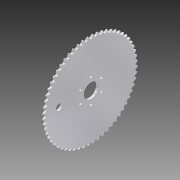
# Autodesk Inventor part: CatapultSprocket
Saved by Autodesk Inventor 2013 (Build 170138000, 138)
## iProperties
Category: iParts
Company: FirstCadLibrary
Shininess: 64.0
Length Units: 11272
Angle Units: 11279
Time Units: 11290
Mass Units: 11286
Length Display Precision: 3
Angle Display Precision: 2
Compacted: True
Part Number: CatapultSprocket
Document SubType Name: Modeling
Created: 2006-02-06
Designer: Ed Sparks
Material: Aluminum-6061
Engineer: Ed Sparks
Density: 7.86 g/cm^3
Density: 0.0
Volumn: 0.0
Area: 0.0
PropertySet Name: Model Information
Control State: 0
Master: False
Checked Out: False
Title: i-Sprocket
Subject: i-Sprocket
Author: Ed Sparks
Keywords: Sprocket
Autodesk Inventor part; units mm, degrees
ref_plane "YZ Plane" through (0, 0, 0) normal (1, 0, 0) x (0, 1, 0)
ref_plane "XZ Plane" through (0, 0, 0) normal (0, 1, 0) x (-1, 0, 0)
ref_plane "XY Plane" through (0, 0, 0) normal (0, 0, 1) x (1, 0, 0)
sketch "Sketch1" plane through (0, 0, 0) normal (0, 0, 1) x (1, 0, 0)
  line L0 (-2.1384, 0) -> (2.1384, 0)
  line L1 (0, 0) -> (0, 93.7314) construction
  line L2 (-0.9484, 93.7314) -> (0.9484, 93.7314)
  line L3 (-2.1384, 0) -> (-2.1384, 88.9689)
  line L4 (2.1384, 0) -> (2.1384, 88.9689)
  arc A0 (-0.9484, 93.7314) -> (-2.1384, 88.9689) centre (7.9867, 88.9689) ccw
  arc A1 (2.1384, 88.9689) -> (0.9484, 93.7314) centre (-7.9867, 88.9689) ccw
  point P0 (25.317, 18.8926)
  dimension "d0" = 4.2767
  dimension "d1" = 93.7314
  dimension "d2" = 4.7625
  dimension "d3" = 10.1251
  constraints: 10 end point, 4 point on circle, 2 centre point, 2 coincident, 2 horizontal, 2 horizontal alignment, 2 midpoint, 2 parallel, 2 perpendicular, 2 symmetric about line, 1 other
  measures "d0" distance of L0.start L0.end
  measures "d1" distance between parallel lines of L0 L2
  measures "d2" distance from line of point (7.987, 88.969) L2
  measures "d3" distance of point (7.987, 88.969) L3.end
revolve "Sprocket Blank" add sketch "Sketch1" angle 360 about axis through (-2.1384, 0, 0) along (1, 0, 0)
sketch "Sketch2" plane through (2.1384, 0, 0) normal (1, 0, 0) x (0, 0, -1)
  circle A0 centre (0, 0) radius 88.9689 projected
  line L0 (0, 0) -> (0, 35.1967) construction
  circle A1 centre (0, 0) radius 90.9986 construction
  line L1 (0, 0) -> (1.8934, 36.1291) construction
  arc A2 (-2.096, 89.4758) -> (2.096, 89.4758) centre (0, 90.9986) ccw
  arc A3 (2.096, 89.4758) -> (3.1421, 91.672) centre (-3.2878, 93.3874) ccw
  arc A4 (-3.1421, 91.672) -> (-2.096, 89.4758) centre (3.2878, 93.3874) ccw
  line L2 (0, 0) -> (-1.8265, 34.8524) construction
  arc A5 (-3.1421, 91.672) -> (-4.9302, 94.0746) centre (-7.0515, 90.6291) ccw
  arc A6 (4.9302, 94.0746) -> (3.1421, 91.672) centre (7.0515, 90.6291) ccw
  arc A7 (4.9302, 94.0746) -> (-4.9302, 94.0746) centre (0, 0) ccw
  dimension "d9" = 181.9973
  dimension "d10" = 3
  dimension "d11" = 7.0515
  dimension "d12" = 3.2879
  dimension "d13" = 0.3695
  dimension "d15" = 2.3888
  dimension "d17" = 5.1816
  constraints: 14 coincident, 12 point on circle, 6 centre point, 6 end point, 3 point on line, 3 tangent, 2 horizontal alignment, 2 symmetric about line, 1 vertical, 1 vertical alignment, 5 other
  measures "d10" angle of L1 L0
  measures "d11" horizontal distance of point (7.052, 90.629) L0.start
  measures "d12" horizontal distance of point (-3.288, 93.387) L0.start
  measures "d13" vertical distance of point (7.052, 90.629) point (0, 90.999)
  measures "d15" vertical distance of point (0, 90.999) point (-3.288, 93.387)
  measures "d17" diameter of A2
extrude "Tooth Profile" cut sketch "Sketch2" against normal blind 25.4 contours A2 A0 | A0 A2 A4 A5 A7 A6 A3 picked at (0, 88.7808)
sketch "Sketch5" plane through (-2.1384, 0, 0) normal (-1, 0, 0) x (0, 0, 1)
  circle A0 centre (0, 0) radius 88.9689 projected
  constraints: 1 coincident
hole "Bore" at (-2.1384, 0, 0) direction (1, 0, 0) diameter 28.5623 end through all
pattern_circular "Circular Pattern2" count 60 over 360 about axis through (-10, 0, 0) along (1, 0, 0) of "Tooth Profile"
sketch "Sketch10" plane through (2.1384, 90.9986, 0) normal (1, 0, 0) x (0, 0, -1)
  arc A0 (-71.0301, -144.5728) -> (1.592, -2.044) centre (0, -90.9986) ccw projected
  line L0 (0, -90.9986) -> (0, -46.364) construction
  point P0 (0, -67.1861)
  dimension "d56" = 23.8125
  constraints: 2 end point, 1 coincident, 1 point on line, 1 vertical
  measures "d56" distance of point (0, -67.186) A0.centre
hole "Hole3" at (2.1384, 23.8125, 0) direction (-1, 0, 0) diameter 5.2324 end through all
pattern_circular "Circular Pattern3" count 6 over 360 about axis through (262.9377, 0, 0) along (-1, 0, 0) of "Hole3"
sketch "Sketch11" plane through (2.1384, 0, 0) normal (1, 0, 0) x (0, -0.0523, -0.9986)
  circle A0 centre (0, 0) radius 14.2811 projected
  line L0 (0, 0) -> (-63.5, 0) construction
  line L1 (0, 0) -> (63.5, 0) construction
  dimension "d67" = 63.5
  dimension "d68" = 180
  constraints: 4 end point, 2 horizontal, 1 coincident, 1 collinear
  measures "d67" distance of L0.start L0.end
  measures "d68" angle of L0 L1
hole "Hole4" at (2.1384, 3.3233, 63.413) direction (-1, 0, 0) diameter 12.7 end through all
equation "\"d0\" = Sprocket_Thickness"
equation "\"d1\" = Outside_Radius"
equation "\"d2\" = Depth_Of_Chamfer"
equation "\"d3\" = Chamfer_Radius"
equation "\"d9\" = Pitch_Diameter"
equation "\"d11\" = W_"
equation "\"d12\" = M_"
equation "\"d13\" = V_"
equation "\"d15\" = T_"
equation "\"d17\" = Seating_Curve_Diameter"
equation "\"d42\" = Bore_Diameter"
equation "\"Chamfer_Radius\" = 1.063 * Chain_Pitch"
equation "\"Depth_Of_Chamfer\" = 0.5 * Chain_Pitch"
equation "\"Chain_Pitch\" = 9.525"
equation "\"Roller_Diameter\" = 5.08"
equation "\"d14\" = F_"
equation "\"d16\" = E_"
equation "\"Hub_Diameter\" = 37.30625"
equation "\"Bore_Diameter\" = 28.5623"
equation "\"Length_Through_Bore\" = 19.05"
equation "\"Key_Width\" = 3.175"
equation "\"Hub_Chamfer\" = 0.254"
equation "\"Sprocket_Thickness\" = 4.276725"
equation "\"Outside_Radius\" = 93.731413"
equation "\"Pitch_Diameter\" = 181.997248"
equation "\"Seating_Curve_Diameter\" = 5.1816"
equation "\"F_\" = 4.069007"
equation "\"E_\" = 6.6548"
equation "\"W_\" = 7.051523"
equation "\"M_\" = 3.287845"
equation "\"V_\" = 0.369555"
equation "\"T_\" = 2.388759"
body "Solid1"
